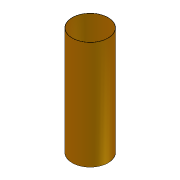
# Autodesk Inventor part: kapton_wrap_battery
Saved by Autodesk Inventor 2014 SP1 (Build 180222100, 222)
## iProperties
Created: 2013-03-29
Part Number: kapton_wrap_battery
Document SubType Name: Modeling
Designer: Robert Davis
Density: 1.425 g/cm^3
Material: Acetal Resin, Black
Mass: 0.382065 g
Surface Area: 53.7288 cm^2
Volume: 0.268116 cm^3
Appearance: Orange (Dark)
Author: Robert Davis
Autodesk Inventor part; units mm, degrees
ref_plane "YZ Plane" through (0, 0, 0) normal (1, 0, 0) x (0, 1, 0)
ref_plane "XZ Plane" through (0, 0, 0) normal (0, 1, 0) x (-1, 0, 0)
ref_plane "XY Plane" through (0, 0, 0) normal (0, 0, 1) x (1, 0, 0)
sketch "Sketch1" plane through (0, 0, 0) normal (0, 0, 1) x (1, 0, 0)
  circle A0 centre (0, 0) radius 8.35
  circle A1 centre (0, 0) radius 8.45
  dimension "d0" = 16.7
  dimension "d1" = 0.1
  constraints: 2 centre point, 1 coincident
  measures "d0" diameter of A0
  measures "d1" radial gap between concentric circles of A1 A0
extrude "Extrusion1" add sketch "Sketch1" along normal mid plane 50.8
body "Solid1"
